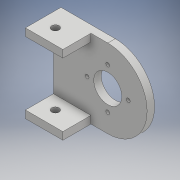
# Autodesk Inventor part: BaseJointMotorMount
Saved by Autodesk Inventor 2018 (Build 220112000, 112)
## iProperties
Created: 2017-05-31
Part Number: BaseJointMotorMount
Material: Generic
Document SubType Name: Modeling
Designer: Damian
Density: 1 g/cm^3
Appearance: Default
Author: Damian
Autodesk Inventor part; units mm, degrees
ref_plane "YZ Plane" through (0, 0, 0) normal (1, 0, 0) x (0, 1, 0)
ref_plane "XZ Plane" through (0, 0, 0) normal (0, 1, 0) x (-1, 0, 0)
ref_plane "XY Plane" through (0, 0, 0) normal (0, 0, 1) x (1, 0, 0)
sketch "Sketch1" plane through (0, 0, 0) normal (1, 0, 0) x (0, 1, 0)
  line L0 (0, 25.9556) -> (0, 21.9556)
  line L1 (0, 21.9556) -> (15, 21.9556)
  line L2 (15, 21.9556) -> (15, -12.0444)
  line L3 (15, -12.0444) -> (0, -12.0444)
  line L4 (0, -12.0444) -> (0, -16.0444)
  line L5 (0, -16.0444) -> (19, -16.0444)
  line L6 (19, -16.0444) -> (19, 25.9556)
  line L7 (19, 25.9556) -> (0, 25.9556)
  point P0 (0, 0)
  dimension "d0" = 4
  dimension "d1" = 4
  dimension "d2" = 15
  dimension "d3" = 42
  constraints: 16 end point, 6 perpendicular, 2 point on line, 1 collinear, 1 vertical
  measures "d0" distance of L3.end L4.end
  measures "d1" horizontal distance of L5.end L2.end
  measures "d2" distance of L2.end L3.end
  measures "d3" distance of L5.end L6.end
extrude "Extrusion1" add sketch "Sketch1" along normal blind 50
sketch "Sketch2" plane through (0, 0, 25.9556) normal (0, 0, 1) x (1, 0, 0)
  line L0 (50, 0) -> (20, 0)
  line L1 (20, 0) -> (20, 15)
  line L2 (20, 15) -> (50, 15)
  line L3 (50, 15) -> (50, 0)
  point P0 (0, 0)
  dimension "d6" = 15
  dimension "d7" = 30
  constraints: 8 end point, 2 parallel, 1 horizontal, 1 perpendicular
  measures "d6" distance of L2.end L0.start
  measures "d7" distance of L1.end L2.end
extrude "Extrusion2" cut sketch "Sketch2" against normal blind 50
fillet "Fillet1" radius 21 2 edges at (50, 17, 25.9556) (50, 17, -16.0444)
hole "Hole1" at (29, 19, 4.9556) direction (0, -1, 0) diameter 15 depth 8 tip angle 118
hole "Hole2" at (29, 19, -6.0444) direction (0, -1, 0) diameter 2 depth 8 tip angle 118
hole "Hole6" at (8, 8, -16.0444) direction (0, 0, 1) diameter 4 depth 42
pattern_circular "Circular Pattern1" count 4 over 360 about axis through (29, 15, 4.9556) along (0, 1, 0) of "Hole2"
body "Solid1"
